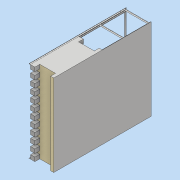
# Autodesk Inventor part: Khung đỡ
Saved by Autodesk Inventor 2018 (Build 220112000, 112)
## iProperties
Created: 2020-08-07
Part Number: Khung đỡ
Material: Generic
Document SubType Name: Modeling
Designer: ASUS
Density: 1 g/cm^3
Appearance: Default
Author: ASUS
Autodesk Inventor part; units mm, degrees
ref_plane "YZ Plane" through (0, 0, 0) normal (1, 0, 0) x (0, 1, 0)
ref_plane "XZ Plane" through (0, 0, 0) normal (0, 1, 0) x (-1, 0, 0)
ref_plane "XY Plane" through (0, 0, 0) normal (0, 0, 1) x (1, 0, 0)
sketch "Sketch1" plane through (0, 0, 0) normal (0, 1, 0) x (-1, 0, 0)
  line L0 (0, 0) -> (60, 0)
  line L1 (60, 0) -> (60, 0)
  line L2 (55, -5) -> (13, -5)
  line L3 (0, -5) -> (0, 0)
  line L4 (0, 0) -> (5, 0)
  line L5 (5, -13) -> (5, -56)
  line L6 (1, -60) -> (0, -60)
  line L7 (0, -60) -> (0, 0)
  arc A0 (13, -5) -> (5, -13) centre (13, -13) ccw
  arc A1 (55, -5) -> (60, 0) centre (55, 0) ccw
  arc A2 (1, -60) -> (5, -56) centre (1, -56) ccw
  line L8 (0, -1435) -> (312.5963, -1435)
  line L9 (0, -2870) -> (60, -2870)
  line L10 (60, -2870) -> (60, -2870)
  line L11 (55, -2865) -> (13, -2865)
  line L12 (0, -2865) -> (0, -2870)
  line L13 (0, -2870) -> (5, -2870)
  line L14 (5, -2857) -> (5, -2814)
  line L15 (1, -2810) -> (0, -2810)
  line L16 (0, -2810) -> (0, -2870)
  arc A3 (5, -2857) -> (13, -2865) centre (13, -2857) ccw
  arc A4 (60, -2870) -> (55, -2865) centre (55, -2870) ccw
  arc A5 (5, -2814) -> (1, -2810) centre (1, -2814) ccw
  line L17 (5, -1640) -> (0, -1640)
  line L18 (0, -1627) -> (0, -1585)
  line L19 (5, -1580) -> (5, -1580)
  line L20 (5, -1580) -> (5, -1640)
  line L21 (5, -1640) -> (-55, -1640)
  line L22 (-55, -1640) -> (-55, -1640)
  line L23 (-50, -1635) -> (-8, -1635)
  line L24 (5, -1635) -> (5, -1640)
  arc A6 (-8, -1635) -> (0, -1627) centre (-8, -1627) ccw
  arc A7 (5, -1580) -> (0, -1585) centre (5, -1585) ccw
  arc A8 (-50, -1635) -> (-55, -1640) centre (-50, -1640) ccw
  point P0 (60, -5)
  point P1 (5, -60)
  point P2 (60, -2865)
  point P3 (5, -2810)
  point P4 (0, -1580)
  point P5 (-55, -1635)
  dimension "d1" = 60
  dimension "d2" = 5
  dimension "d3" = 5
  dimension "d4" = 60
  dimension "d5" = 8
  dimension "d6" = 5
  dimension "d7" = 4
  dimension "d8" = 1435
  dimension "d11" = 5
  dimension "d12" = 60
  dimension "d13" = 1290
  dimension "d14" = 60
  dimension "d15" = 5
  dimension "d16" = 8
  dimension "d17" = 5
  dimension "d38" = 0
  constraints: 50 end point, 18 point on circle, 18 point on line, 16 symmetric about line, 12 tangent, 9 centre point, 8 parallel, 5 horizontal, 4 perpendicular, 1 equal radius, 3 other
  measures "d1" distance of point (60, -5) L3.start
  measures "d2" distance of L0.end point (60, -5)
  measures "d3" distance of point (5, -60) L6.end
  measures "d4" distance of L4.end point (5, -60)
  measures "d5" radius of A0
  measures "d6" radius of A1
  measures "d7" radius of A2
  measures "d8" distance from line of L0.start L8
  measures "d11" distance of point (0, -1580) L19.end
  measures "d12" distance of L17.end point (0, -1580)
  measures "d13" distance between parallel lines of L9 L19
  measures "d14" distance of point (-55, -1635) L24.start
  measures "d15" distance of L21.end point (-55, -1635)
  measures "d16" radius of A6
  measures "d17" radius of A7
  measures "d38" distance between parallel lines of L14 L20
extrude "Extrusion1" add sketch "Sketch1" along normal blind 3350
sketch "Sketch5" plane through (-60, 0, -2870) normal (0, 0, -1) x (-1, 0, 0)
  line L0 (-60, 3350) -> (0, 3350) projected
  line L1 (0, 3350) -> (-60, 3350)
  line L2 (-60, 3350) -> (-60, 3350)
  line L3 (-55, 3355) -> (-13, 3355)
  line L4 (0, 3355) -> (0, 3350)
  line L5 (0, 3355) -> (-5, 3355)
  line L6 (-5, 3363) -> (-5, 3405)
  line L7 (0, 3410) -> (0, 3410)
  line L8 (0, 3410) -> (0, 3355)
  arc A0 (-13, 3355) -> (-5, 3363) centre (-13, 3363) ccw
  arc A1 (0, 3410) -> (-5, 3405) centre (0, 3405) ccw
  arc A2 (-55, 3355) -> (-60, 3350) centre (-55, 3350) ccw
  point P0 (-60, 0)
  point P1 (-60, 3355)
  point P2 (-5, 3410)
  dimension "d84" = 60
  dimension "d85" = 5
  dimension "d86" = 5
  dimension "d87" = 55
  dimension "d88" = 8
  dimension "d89" = 5
  constraints: 16 end point, 6 point on circle, 6 point on line, 6 tangent, 4 parallel, 3 centre point, 2 horizontal, 2 perpendicular, 1 equal radius
  measures "d84" distance of point (-60, 3355) L4.start
  measures "d85" distance of L1.end point (-60, 3355)
  measures "d86" distance of point (-5, 3410) L7.end
  measures "d87" distance of L5.end point (-5, 3410)
  measures "d88" radius of A0
  measures "d89" radius of A1
extrude "Extrusion3" add sketch "Sketch5" against normal blind 2870
sketch "Sketch6" plane through (0, 0, -2870) normal (1, 0, 0) x (0, 0, -1)
  line L0 (0, 0) -> (0, 3350) projected
  line L1 (0, 3350) -> (-60, 3350)
  line L2 (-60, 3350) -> (-60, 3350)
  line L3 (-55, 3345) -> (-13, 3345)
  line L4 (0, 3345) -> (0, 3350)
  line L5 (0, 3345) -> (-5, 3345)
  line L6 (-5, 3337) -> (-5, 3295)
  line L7 (0, 3290) -> (0, 3290)
  line L8 (0, 3290) -> (0, 3345)
  arc A0 (-5, 3337) -> (-13, 3345) centre (-13, 3337) ccw
  arc A1 (-60, 3350) -> (-55, 3345) centre (-55, 3350) ccw
  arc A2 (-5, 3295) -> (0, 3290) centre (0, 3295) ccw
  line L9 (0, 2450) -> (-60, 2450)
  line L10 (-60, 2450) -> (-60, 2450)
  line L11 (-55, 2445) -> (-13, 2445)
  line L12 (0, 2445) -> (0, 2450)
  line L13 (-60, 3350) -> (-1230, 3350) projected
  line L14 (0, 2445) -> (-5, 2445)
  line L15 (-5, 2437) -> (-5, 2395)
  line L16 (0, 2390) -> (0, 2390)
  line L17 (0, 2390) -> (0, 2445)
  arc A3 (-5, 2437) -> (-13, 2445) centre (-13, 2437) ccw
  arc A4 (-5, 2395) -> (0, 2390) centre (0, 2395) ccw
  arc A5 (-60, 2450) -> (-55, 2445) centre (-55, 2450) ccw
  line L18 (-1230, 0) -> (-1230, 3350) projected
  line L19 (-1230, 3350) -> (-1290, 3350)
  line L20 (-1290, 3350) -> (-1290, 3350)
  line L21 (-1285, 3345) -> (-1243, 3345)
  line L22 (-1230, 3345) -> (-1230, 3350)
  line L23 (-1230, 3345) -> (-1235, 3345)
  line L24 (-1235, 3337) -> (-1235, 3295)
  line L25 (-1230, 3290) -> (-1230, 3290)
  line L26 (-1230, 3290) -> (-1230, 3345)
  arc A6 (-1290, 3350) -> (-1285, 3345) centre (-1285, 3350) ccw
  arc A7 (-1235, 3295) -> (-1230, 3290) centre (-1230, 3295) ccw
  arc A8 (-1235, 3337) -> (-1243, 3345) centre (-1243, 3337) ccw
  line L27 (-1290, 0) -> (-1290, 3350) projected
  line L28 (-1230, 2450) -> (-1290, 2450)
  line L29 (-1290, 2450) -> (-1290, 2450)
  line L30 (-1285, 2445) -> (-1243, 2445)
  line L31 (-1230, 2445) -> (-1230, 2450)
  line L32 (-1230, 2445) -> (-1235, 2445)
  line L33 (-1235, 2437) -> (-1235, 2395)
  line L34 (-1230, 2390) -> (-1230, 2390)
  line L35 (-1230, 2390) -> (-1230, 2445)
  arc A9 (-1235, 2437) -> (-1243, 2445) centre (-1243, 2437) ccw
  arc A10 (-1235, 2395) -> (-1230, 2390) centre (-1230, 2395) ccw
  arc A11 (-1290, 2450) -> (-1285, 2445) centre (-1285, 2450) ccw
  line L36 (-2865, 3350) -> (-2870, 3350) projected
  line L37 (-2870, 3350) -> (-2810, 3350)
  line L38 (-2810, 3350) -> (-2810, 3350)
  line L39 (-2815, 3345) -> (-2857, 3345)
  line L40 (-2870, 3345) -> (-2870, 3350)
  line L41 (-2870, 3345) -> (-2865, 3345)
  line L42 (-2865, 3337) -> (-2865, 3295)
  line L43 (-2870, 3290) -> (-2870, 3290)
  line L44 (-2870, 3290) -> (-2870, 3345)
  arc A12 (-2870, 3290) -> (-2865, 3295) centre (-2870, 3295) ccw
  arc A13 (-2815, 3345) -> (-2810, 3350) centre (-2815, 3350) ccw
  arc A14 (-2857, 3345) -> (-2865, 3337) centre (-2857, 3337) ccw
  line L45 (-2810, 2450) -> (-2870, 2450)
  line L46 (-2870, 2450) -> (-2870, 2445)
  line L47 (-2857, 2445) -> (-2815, 2445)
  line L48 (-2810, 2450) -> (-2810, 2450)
  line L49 (-1285, 3350) -> (-2810, 3350) projected
  line L50 (-2870, 2445) -> (-2865, 2445)
  line L51 (-2865, 2437) -> (-2865, 2395)
  line L52 (-2870, 2390) -> (-2870, 2390)
  line L53 (-2870, 2390) -> (-2870, 2445)
  arc A15 (-2857, 2445) -> (-2865, 2437) centre (-2857, 2437) ccw
  arc A16 (-2815, 2445) -> (-2810, 2450) centre (-2815, 2450) ccw
  arc A17 (-2870, 2390) -> (-2865, 2395) centre (-2870, 2395) ccw
  point P0 (-2870, 0)
  point P1 (-60, 3345)
  point P2 (-5, 3290)
  point P3 (-60, 2445)
  point P4 (-5, 2390)
  point P5 (-1290, 3345)
  point P6 (-1235, 3290)
  point P7 (-1290, 2445)
  point P8 (-1235, 2390)
  point P9 (-2810, 3345)
  point P10 (-2865, 3290)
  point P11 (-2810, 2445)
  point P12 (-2865, 2390)
  dimension "d92" = 60
  dimension "d93" = 5
  dimension "d94" = 5
  dimension "d95" = 55
  dimension "d96" = 8
  dimension "d97" = 5
  dimension "d98" = 60
  dimension "d99" = 5
  dimension "d100" = 900
  dimension "d101" = 5
  dimension "d102" = 55
  dimension "d103" = 8
  dimension "d104" = 5
  dimension "d105" = 60
  dimension "d106" = 5
  dimension "d107" = 5
  dimension "d108" = 55
  dimension "d109" = 5
  dimension "d110" = 8
  dimension "d111" = 5
  dimension "d112" = 900
  dimension "d113" = 5
  dimension "d114" = 55
  dimension "d115" = 8
  dimension "d116" = 5
  dimension "d117" = 60
  dimension "d118" = 5
  dimension "d119" = 5
  dimension "d120" = 55
  dimension "d121" = 5
  dimension "d122" = 8
  dimension "d123" = 60
  dimension "d124" = 5
  dimension "d125" = 900
  dimension "d126" = 5
  dimension "d127" = 55
  dimension "d128" = 8
  dimension "d129" = 5
  constraints: 96 end point, 39 point on line, 36 point on circle, 36 tangent, 24 parallel, 18 centre point, 12 horizontal, 12 perpendicular, 6 equal radius
  measures "d92" distance of L4.start point (-60, 3345)
  measures "d93" distance of point (-60, 3345) L1.end
  measures "d94" distance of L7.end point (-5, 3290)
  measures "d95" distance of point (-5, 3290) L5.end
  measures "d96" radius of A0
  measures "d97" radius of A1
  measures "d98" distance of L12.start point (-60, 2445)
  measures "d99" distance of point (-60, 2445) L9.end
  measures "d100" distance between parallel lines of L13 L9
  measures "d101" distance of L16.end point (-5, 2390)
  measures "d102" distance of point (-5, 2390) L14.end
  measures "d103" radius of A3
  measures "d104" radius of A4
  measures "d105" distance of L22.start point (-1290, 3345)
  measures "d106" distance of point (-1290, 3345) L19.end
  measures "d107" distance of L25.end point (-1235, 3290)
  measures "d108" distance of point (-1235, 3290) L23.end
  measures "d109" radius of A6
  measures "d110" radius of A8
  measures "d111" distance of point (-1290, 2445) L28.end
  measures "d112" distance between parallel lines of L13 L28
  measures "d113" distance of L34.end point (-1235, 2390)
  measures "d114" distance of point (-1235, 2390) L32.end
  measures "d115" radius of A9
  measures "d116" radius of A10
  measures "d117" distance of point (-2810, 3345) L40.start
  measures "d118" distance of L37.end point (-2810, 3345)
  measures "d119" distance of point (-2865, 3290) L43.end
  measures "d120" distance of L41.end point (-2865, 3290)
  measures "d121" radius of A12
  measures "d122" radius of A14
  measures "d123" distance of point (-2810, 2445) L46.end
  measures "d124" distance of L46.end L45.end
  measures "d125" distance between parallel lines of L49 L45
  measures "d126" distance of point (-2865, 2390) L52.end
  measures "d127" distance of L50.end point (-2865, 2390)
  measures "d128" radius of A15
  measures "d129" radius of A16
extrude "Extrusion4" add sketch "Sketch6" along normal blind 800 contours A4 L15 A3 L11 A5 L9 L0 | A13 L39 A14 L42 A12 L44 L40 L36 L37 | L18 A7 L24 A8 L21 A6 L19 | A2 L6 A0 L3 A1 L1 L0 | L18 A10 L33 A9 L30 A11 L28 | A16 L47 A15 L51 A17 L53 L46 L45
sketch "Sketch7" plane through (0, 0, -2810) normal (1, 0, 0) x (0, 0, -1)
  line L0 (60, 0) -> (60, 3350) projected
  line L1 (-2810, 0) -> (-2810, 3350) projected
  line L2 (60, 1530) -> (-2810, 1530)
  line L3 (-2810, 1530) -> (-2810, 1390)
  line L4 (-2810, 1390) -> (60, 1390)
  line L5 (60, 1390) -> (60, 1530)
  line L6 (-1230, 3350) -> (-2750, 3350) projected
  line L7 (60, 170) -> (-2810, 170)
  line L8 (-2810, 170) -> (-2810, 310)
  line L9 (-2810, 310) -> (60, 310)
  line L10 (60, 310) -> (60, 170)
  line L11 (60, 1530) -> (-80, 1530)
  line L12 (-80, 1530) -> (-80, 170)
  line L13 (-80, 170) -> (60, 170)
  line L14 (60, 170) -> (60, 1530)
  line L15 (-2810, 1530) -> (-2670, 1530)
  line L16 (-2670, 1530) -> (-2670, 170)
  line L17 (-2670, 170) -> (-2810, 170)
  line L18 (-2810, 170) -> (-2810, 1530)
  dimension "d132" = 140
  dimension "d133" = 1820
  dimension "d134" = 140
  dimension "d135" = 170
  dimension "d137" = 140
  dimension "d138" = 140
  constraints: 32 end point, 8 parallel, 6 point on line, 4 horizontal, 4 perpendicular
  measures "d132" distance of L3.end L2.end
  measures "d133" distance between parallel lines of L6 L2
  measures "d134" distance of L7.end L8.end
  measures "d135" distance from line of L0.start L7
  measures "d137" distance of L13.end L12.end
  measures "d138" distance of L16.end L17.end
extrude "Extrusion5" add sketch "Sketch7" along normal blind 800 contours L7 L12 L9 L0 | L9 L12 L4 L0 | L7 L16 L9 L12 | L4 L12 L2 L0 | L7 L1 L9 L16 | L4 L16 L2 L12 | L9 L1 L4 L16 | L4 L1 L2 L16
sketch "Sketch8" plane through (0, 0, -2810) normal (-1, 0, 0) x (0, 0, 1)
  line L0 (2810, 0) -> (2810, 3350) projected
  line L1 (2810, 0) -> (2670, 0)
  line L2 (2670, 0) -> (2670, 1700)
  line L3 (2670, 1700) -> (2810, 1700)
  line L4 (2810, 1700) -> (2810, 0)
  line L5 (-60, 0) -> (-60, 3350) projected
  line L6 (-60, 0) -> (80, 0)
  line L7 (80, 0) -> (80, 1700)
  line L8 (80, 1700) -> (-60, 1700)
  line L9 (-60, 1700) -> (-60, 0)
  line L10 (328, 1700) -> (188, 1700)
  line L11 (188, 1700) -> (188, 0)
  line L12 (188, 0) -> (328, 0)
  line L13 (328, 0) -> (328, 1700)
  line L14 (436, 1700) -> (576, 1700)
  line L15 (576, 1700) -> (576, 0)
  line L16 (576, 0) -> (436, 0)
  line L17 (436, 0) -> (436, 1700)
  line L18 (824, 1700) -> (684, 1700)
  line L19 (684, 1700) -> (684, 0)
  line L20 (684, 0) -> (824, 0)
  line L21 (824, 0) -> (824, 1700)
  line L22 (1072, 1700) -> (932, 1700)
  line L23 (932, 1700) -> (932, 0)
  line L24 (932, 0) -> (1072, 0)
  line L25 (1072, 0) -> (1072, 1700)
  line L26 (1318, 1700) -> (1178, 1700)
  line L27 (1178, 1700) -> (1178, 0)
  line L28 (1178, 0) -> (1318, 0)
  line L29 (1318, 0) -> (1318, 1700)
  line L30 (1566, 1700) -> (1426, 1700)
  line L31 (1426, 1700) -> (1426, 0)
  line L32 (1426, 0) -> (1566, 0)
  line L33 (1566, 0) -> (1566, 1700)
  line L34 (1814, 1700) -> (1674, 1700)
  line L35 (1674, 1700) -> (1674, 0)
  line L36 (1674, 0) -> (1814, 0)
  line L37 (1814, 0) -> (1814, 1700)
  line L38 (2062, 1700) -> (1922, 1700)
  line L39 (1922, 1700) -> (1922, 0)
  line L40 (1922, 0) -> (2062, 0)
  line L41 (2062, 0) -> (2062, 1700)
  line L42 (2310, 1700) -> (2170, 1700)
  line L43 (2170, 1700) -> (2170, 0)
  line L44 (2170, 0) -> (2310, 0)
  line L45 (2310, 0) -> (2310, 1700)
  line L46 (2558, 1700) -> (2418, 1700)
  line L47 (2418, 1700) -> (2418, 0)
  line L48 (2418, 0) -> (2558, 0)
  line L49 (2558, 0) -> (2558, 1700)
  dimension "d143" = 1700
  dimension "d144" = 140
  dimension "d145" = 1700
  dimension "d146" = 140
  dimension "d147" = 108
  dimension "d148" = 140
  dimension "d149" = 108
  dimension "d150" = 140
  dimension "d151" = 108
  dimension "d152" = 140
  dimension "d153" = 108
  dimension "d154" = 140
  dimension "d155" = 106
  dimension "d156" = 140
  dimension "d157" = 108
  dimension "d158" = 140
  dimension "d159" = 108
  dimension "d160" = 140
  dimension "d161" = 1700
  dimension "d162" = 108
  dimension "d163" = 140
  dimension "d164" = 1700
  dimension "d165" = 108
  dimension "d166" = 140
  dimension "d167" = 108
  dimension "d168" = 140
  constraints: 96 end point, 24 parallel, 12 horizontal, 12 perpendicular
  measures "d143" distance of L1.end L2.end
  measures "d144" distance of L8.end L7.end
  measures "d145" distance of L7.end L6.end
  measures "d146" distance of L12.end L11.end
  measures "d147" distance between parallel lines of L7 L11
  measures "d148" distance of L15.end L16.end
  measures "d149" distance between parallel lines of L13 L17
  measures "d150" distance of L20.end L19.end
  measures "d151" distance between parallel lines of L15 L19
  measures "d152" distance of L24.end L23.end
  measures "d153" distance between parallel lines of L21 L23
  measures "d154" distance of L28.end L27.end
  measures "d155" distance between parallel lines of L27 L25
  measures "d156" distance of L32.end L31.end
  measures "d157" distance between parallel lines of L31 L29
  measures "d158" distance of L36.end L35.end
  measures "d159" distance between parallel lines of L33 L35
  measures "d160" distance of L40.end L39.end
  measures "d161" distance of L39.end L38.end
  measures "d162" distance between parallel lines of L37 L39
  measures "d163" distance of L44.end L43.end
  measures "d164" distance of L43.end L42.end
  measures "d165" distance between parallel lines of L41 L43
  measures "d166" distance of L48.end L47.end
  measures "d167" distance between parallel lines of L45 L47
  measures "d168" distance between parallel lines of L0 L2
extrude "Extrusion6" add sketch "Sketch8" against normal blind 150
sketch "Sketch11" plane through (800, 0, -2810) normal (1, 0, 0) x (0, 0, -1)
  line L0 (60, 3410) -> (-2810, 3410) projected
  line L1 (60, 3410) -> (-2810, 3410)
  line L2 (-2810, 3410) -> (-2810, 0)
  line L3 (-2810, 0) -> (60, 0)
  line L4 (60, 0) -> (60, 3410)
  constraints: 8 end point, 2 parallel, 1 horizontal, 1 perpendicular
extrude "Extrusion7" add sketch "Sketch11" along normal blind 10
sketch "Sketch12" plane through (-60, 0, -2870) normal (0, 0, -1) x (-1, 0, 0)
  line L0 (-860, 2390) -> (-860, 1530) projected
  line L1 (-860, 1530) -> (-760, 1530)
  line L2 (-760, 1530) -> (-760, 1700)
  line L3 (-760, 1700) -> (-860, 1700)
  line L4 (-860, 1700) -> (-860, 1530)
  line L5 (-860, 0) -> (-860, 170) projected
  line L6 (-860, 0) -> (-760, 0)
  line L7 (-760, 0) -> (-760, 170)
  line L8 (-760, 170) -> (-860, 170)
  line L9 (-860, 170) -> (-860, 0)
  point P0 (-60, 0)
  dimension "d173" = 100
  dimension "d174" = 170
  dimension "d175" = 100
  dimension "d176" = 170
  constraints: 16 end point, 4 parallel, 2 horizontal, 2 perpendicular
  measures "d173" distance of L3.end L2.end
  measures "d174" distance of L2.end L1.end
  measures "d175" distance of L8.end L7.end
  measures "d176" distance of L7.end L6.end
extrude "Extrusion8" add sketch "Sketch12" against normal blind 2870
sketch "Sketch13" plane through (-60, 0, -2870) normal (0, 0, -1) x (-1, 0, 0)
  circle A0 centre (-30, 3185) radius 4
  line L0 (-60, 3350) -> (-860, 3350) projected
  point P0 (-60, 0)
  dimension "d179" = 8
  dimension "d180" = 165
  constraints: 1 centre point
  measures "d179" diameter of A0
  measures "d180" distance from line of L0 A0.centre
extrude "Extrusion9" cut sketch "Sketch13" against normal blind 3000
sketch "Sketch16" plane through (-47, 3355, 0) normal (0, 1, 0) x (1, 0, 0)
  circle A0 centre (26, 1657) radius 5
  line L0 (47, 1640) -> (847, 1640) projected
  line L1 (-13, 2870) -> (-13, 0) projected
  point P0 (47, 0)
  dimension "d183" = 10
  dimension "d184" = 17
  dimension "d185" = 39
  constraints: 1 centre point
  measures "d183" diameter of A0
  measures "d184" distance from line of L0 A0.centre
  measures "d185" distance from line of L1 A0.centre
extrude "Extrusion10" cut sketch "Sketch16" against normal blind 10
equation "\"d186\" = d183"
body "Solid1"
